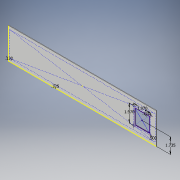
# Autodesk Inventor part: NMT_backpanel
Saved by Autodesk Inventor 2017 (Build 210142000, 142)
## iProperties
Created: 2017-02-15
Part Number: NMT_backpanel
Material: Generic
Document SubType Name: Modeling
Designer: Zara
Density: 1 g/cm^3
Appearance: Default
Author: Zara
Autodesk Inventor part; units mm, degrees
ref_plane "YZ Plane" through (0, 0, 0) normal (1, 0, 0) x (0, 1, 0)
ref_plane "XZ Plane" through (0, 0, 0) normal (0, 1, 0) x (-1, 0, 0)
ref_plane "XY Plane" through (0, 0, 0) normal (0, 0, 1) x (1, 0, 0)
sketch "Sketch1" plane through (0, 0, 0) normal (0, 0, 1) x (1, 0, 0)
  line L0 (-212.471, -44.069) -> (212.471, -44.069)
  line L1 (212.471, -44.069) -> (212.471, 44.069)
  line L2 (212.471, 44.069) -> (-212.471, 44.069)
  line L3 (-212.471, 44.069) -> (-212.471, -44.069)
  line L4 (-212.471, -44.069) -> (212.471, 44.069) construction
  line L5 (212.471, -44.069) -> (-212.471, 44.069) construction
  point P0 (0, 0)
  dimension "d0" = 424.942
  dimension "d1" = 88.138
  constraints: 12 end point, 2 midpoint, 2 parallel, 1 horizontal, 1 perpendicular
  measures "d0" distance of L1.end L2.end
  measures "d1" distance of L0.end L1.end
extrude "Extrusion1" add sketch "Sketch1" along normal blind 1.651
sketch "airflow" plane through (0, 0, 1.651) normal (0, 0, 1) x (1, 0, 0)
  line L0 (146.685, -25.019) -> (196.723, -25.019) construction
  line L1 (196.723, -25.019) -> (196.723, 25.019) construction
  line L2 (196.723, 25.019) -> (146.685, 25.019) construction
  line L3 (146.685, 25.019) -> (146.685, -25.019) construction
  line L4 (146.685, -25.019) -> (196.723, 25.019) construction
  line L5 (196.723, -25.019) -> (146.685, 25.019) construction
  line L6 (-212.471, 44.069) -> (-212.471, -44.069) projected
  line L7 (-212.471, -44.069) -> (212.471, -44.069) projected
  line L8 (-209.423, -35.814) -> (209.423, -35.814) construction
  line L9 (209.423, -35.814) -> (209.423, 35.814) construction
  line L10 (209.423, 35.814) -> (-209.423, 35.814) construction
  line L11 (-209.423, 35.814) -> (-209.423, -35.814) construction
  line L12 (-209.423, -35.814) -> (209.423, 35.814) construction
  line L13 (209.423, -35.814) -> (-209.423, 35.814) construction
  line L14 (150.622, -21.082) -> (192.786, -21.082)
  line L15 (192.786, -21.082) -> (192.786, 21.082)
  line L16 (192.786, 21.082) -> (150.622, 21.082)
  line L17 (150.622, 21.082) -> (150.622, -21.082)
  line L18 (150.622, -21.082) -> (192.786, 21.082) construction
  line L19 (192.786, -21.082) -> (150.622, 21.082) construction
  point P0 (0, 0)
  point P1 (171.704, 0)
  dimension "d4" = 50.038
  dimension "d5" = 50.038
  dimension "d10" = 44.069
  dimension "d11" = 8.255
  dimension "d12" = 3.048
  dimension "d13" = 12.7
  dimension "d14" = 3.937
  constraints: 36 end point, 6 midpoint, 6 parallel, 4 coincident, 3 horizontal, 3 perpendicular, 1 point on line
  measures "d4" distance of L1.end L2.end
  measures "d5" distance of L2.end L0.start
  measures "d10" distance from line of point (171.704, 0) L7
  measures "d11" distance between parallel lines of L8 L7
  measures "d12" distance between parallel lines of L11 L6
  measures "d13" distance between parallel lines of L1 L9
  measures "d14" distance between parallel lines of L2 L16
hole "Hole1" at (196.723, 25.019, 1.651) at (146.685, 25.019, 1.651) at (196.723, -25.019, 1.651) at (146.685, -25.019, 1.651) direction (0, 0, -1) diameter 5.1054 end through all clearance for "Flat Head Machine Screw (82)" size "#10" standard "Ansi Unified Screw Threads"
extrude "Extrusion3" cut sketch "airflow" against normal through all
body "Solid1"
